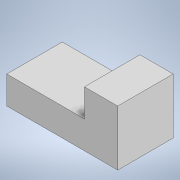
# Autodesk Inventor part: Exercício1.1
Saved by Autodesk Inventor 2022 (Build 260153000, 153)
## iProperties
Created: 2023-03-07
Part Number: Exercício1.1
Material: Genérico
Document SubType Name: Modeling
Designer: jpjoa
Density: 1 g/cm^3
Appearance: Padrão
Author: jpjoa
Autodesk Inventor part; units mm, degrees
ref_plane "YZ Plane" through (0, 0, 0) normal (1, 0, 0) x (0, 1, 0)
ref_plane "XZ Plane" through (0, 0, 0) normal (0, 1, 0) x (-1, 0, 0)
ref_plane "XY Plane" through (0, 0, 0) normal (0, 0, 1) x (1, 0, 0)
sketch "Esboço1" plane through (0, 0, 0) normal (0, 0, 1) x (1, 0, 0)
  line L0 (0, 0) -> (60, 0)
  line L1 (0, 0) -> (60, 0) construction
  line L2 (60, 0) -> (60, 30)
  line L3 (60, 30) -> (42, 30)
  line L4 (0, 0) -> (0, 15)
  line L5 (0, 15) -> (42, 15)
  line L6 (42, 15) -> (42, 30)
  dimension "d0" = 60
  dimension "d2" = 30
  dimension "d3" = 18
  dimension "d4" = 15
  constraints: 14 end point, 4 perpendicular, 2 horizontal, 1 collinear, 1 vertical
  measures "d0" distance of L0.start L0.end
  measures "d2" distance of L1.end L2.end
  measures "d3" distance of L2.end L3.end
  measures "d4" distance of L0.start L4.end
extrude "Extrusão1" add sketch "Esboço1" along normal blind 30
